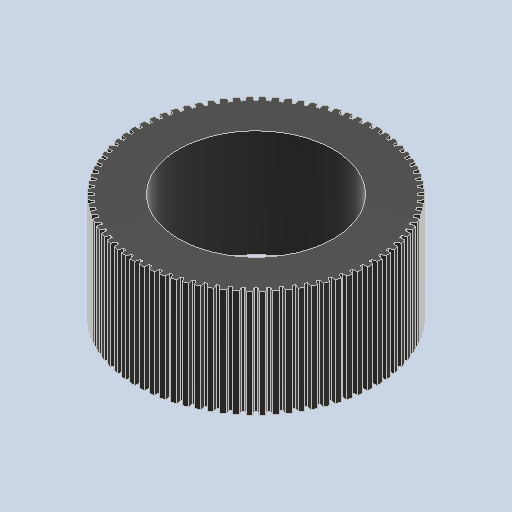
# Autodesk Inventor part: タミヤダンパー3
Saved by Autodesk Inventor 2023 (Build 270158030, 158C)
## iProperties
Part Number: タミヤダンパー3
Material: アセタール樹脂、黒
Document SubType Name: Modeling
Designer: 雪村
Density: 1.425 g/cm^3
Appearance: 滑らか - 黒
Mass: 0.276107 g
Surface Area: 4.29277 cm^2
Volume: 0.193759 cm^3
Author: 雪村
Autodesk Inventor part; units mm, degrees
ref_plane "YZ Plane" through (0, 0, 0) normal (1, 0, 0) x (0, 1, 0)
ref_plane "XZ Plane" through (0, 0, 0) normal (0, 1, 0) x (-1, 0, 0)
ref_plane "XY Plane" through (0, 0, 0) normal (0, 0, 1) x (1, 0, 0)
sketch "スケッチ1" plane through (0, 0, 0) normal (0, 0, 1) x (1, 0, 0)
  circle A0 centre (0, 0) radius 5
  dimension "d0" = 10
  constraints: 1 centre point, 1 coincident
  measures "d0" diameter of A0
extrude "押し出し1" add sketch "スケッチ1" along normal blind 4.5
sketch "スケッチ2" plane through (0, 0, 4.5) normal (0, 0, 1) x (1, 0, 0)
  circle A0 centre (0, 0) radius 3.25
  dimension "d3" = 6.5
  constraints: 1 centre point, 1 coincident
  measures "d3" diameter of A0
extrude "押し出し2" cut sketch "スケッチ2" against normal through all
sketch "スケッチ3" plane through (0, 0, 4.5) normal (0, 0, 1) x (1, 0, 0)
  arc A0 (0.0974, 4.9991) -> (-0.0974, 4.9991) centre (0, 0) ccw
  arc A1 (0.05, 4.8047) -> (-0.05, 4.8047) centre (0, 0) ccw
  line L0 (0.05, 4.8047) -> (0.0974, 4.9991)
  line L1 (-0.05, 4.8047) -> (-0.0974, 4.9991)
  line L2 (0, 4.9011) -> (0, 0)
  line L3 (-0.4268, 4.786) -> (-0.4893, 4.976)
  arc A2 (-0.2952, 4.9913) -> (-0.4893, 4.976) centre (0, 0) ccw
  line L4 (-0.3271, 4.7939) -> (-0.2952, 4.9913)
  arc A3 (-0.3271, 4.7939) -> (-0.4268, 4.786) centre (0, 0) ccw
  line L5 (-0.801, 4.7378) -> (-0.8782, 4.9223)
  arc A4 (-0.6859, 4.9527) -> (-0.8782, 4.9223) centre (0, 0) ccw
  line L6 (-0.7022, 4.7534) -> (-0.6859, 4.9527)
  arc A5 (-0.7022, 4.7534) -> (-0.801, 4.7378) centre (0, 0) ccw
  line L7 (-1.1703, 4.6603) -> (-1.2617, 4.8382)
  arc A6 (-1.0723, 4.8837) -> (-1.2617, 4.8382) centre (0, 0) ccw
  line L8 (-1.073, 4.6837) -> (-1.0723, 4.8837)
  arc A7 (-1.073, 4.6837) -> (-1.1703, 4.6603) centre (0, 0) ccw
  line L9 (-1.5323, 4.5541) -> (-1.6374, 4.7243)
  arc A8 (-1.4522, 4.7845) -> (-1.6374, 4.7243) centre (0, 0) ccw
  line L10 (-1.4372, 4.585) -> (-1.4522, 4.7845)
  arc A9 (-1.4372, 4.585) -> (-1.5323, 4.5541) centre (0, 0) ccw
  line L11 (-1.8849, 4.4199) -> (-2.003, 4.5813)
  arc A10 (-1.8231, 4.6558) -> (-2.003, 4.5813) centre (0, 0) ccw
  line L12 (-1.7925, 4.4581) -> (-1.8231, 4.6558)
  arc A11 (-1.7925, 4.4581) -> (-1.8849, 4.4199) centre (0, 0) ccw
  line L13 (-2.2259, 4.2584) -> (-2.3563, 4.41)
  arc A12 (-2.1828, 4.4984) -> (-2.3563, 4.41) centre (0, 0) ccw
  line L14 (-2.1368, 4.3038) -> (-2.1828, 4.4984)
  arc A13 (-2.1368, 4.3038) -> (-2.2259, 4.2584) centre (0, 0) ccw
  line L15 (-2.5531, 4.0706) -> (-2.695, 4.2115)
  arc A14 (-2.529, 4.3133) -> (-2.695, 4.2115) centre (0, 0) ccw
  line L16 (-2.4678, 4.1228) -> (-2.529, 4.3133)
  arc A15 (-2.4678, 4.1228) -> (-2.5531, 4.0706) centre (0, 0) ccw
  line L17 (-2.8646, 3.8577) -> (-3.0171, 3.9871)
  arc A16 (-2.8596, 4.1015) -> (-3.0171, 3.9871) centre (0, 0) ccw
  line L18 (-2.7837, 3.9165) -> (-2.8596, 4.1015)
  arc A17 (-2.7837, 3.9165) -> (-2.8646, 3.8577) centre (0, 0) ccw
  line L19 (-3.1584, 3.6211) -> (-3.3207, 3.7381)
  arc A18 (-3.1726, 3.8645) -> (-3.3207, 3.7381) centre (0, 0) ccw
  line L20 (-3.0824, 3.686) -> (-3.1726, 3.8645)
  arc A19 (-3.0824, 3.686) -> (-3.1584, 3.6211) centre (0, 0) ccw
  line L21 (-3.4328, 3.3621) -> (-3.6037, 3.466)
  arc A20 (-3.466, 3.6037) -> (-3.6037, 3.466) centre (0, 0) ccw
  line L22 (-3.3621, 3.4328) -> (-3.466, 3.6037)
  arc A21 (-3.3621, 3.4328) -> (-3.4328, 3.3621) centre (0, 0) ccw
  line L23 (-3.686, 3.0824) -> (-3.8645, 3.1726)
  arc A22 (-3.7381, 3.3207) -> (-3.8645, 3.1726) centre (0, 0) ccw
  line L24 (-3.6211, 3.1584) -> (-3.7381, 3.3207)
  arc A23 (-3.6211, 3.1584) -> (-3.686, 3.0824) centre (0, 0) ccw
  line L25 (-3.9165, 2.7837) -> (-4.1015, 2.8596)
  arc A24 (-3.9871, 3.0171) -> (-4.1015, 2.8596) centre (0, 0) ccw
  line L26 (-3.8577, 2.8646) -> (-3.9871, 3.0171)
  arc A25 (-3.8577, 2.8646) -> (-3.9165, 2.7837) centre (0, 0) ccw
  line L27 (-4.1228, 2.4678) -> (-4.3133, 2.529)
  arc A26 (-4.2115, 2.695) -> (-4.3133, 2.529) centre (0, 0) ccw
  line L28 (-4.0706, 2.5531) -> (-4.2115, 2.695)
  arc A27 (-4.0706, 2.5531) -> (-4.1228, 2.4678) centre (0, 0) ccw
  line L29 (-4.3038, 2.1368) -> (-4.4984, 2.1828)
  arc A28 (-4.41, 2.3563) -> (-4.4984, 2.1828) centre (0, 0) ccw
  line L30 (-4.2584, 2.2259) -> (-4.41, 2.3563)
  arc A29 (-4.2584, 2.2259) -> (-4.3038, 2.1368) centre (0, 0) ccw
  line L31 (-4.4581, 1.7925) -> (-4.6558, 1.8231)
  arc A30 (-4.5813, 2.003) -> (-4.6558, 1.8231) centre (0, 0) ccw
  line L32 (-4.4199, 1.8849) -> (-4.5813, 2.003)
  arc A31 (-4.4199, 1.8849) -> (-4.4581, 1.7925) centre (0, 0) ccw
  line L33 (-4.585, 1.4372) -> (-4.7845, 1.4522)
  arc A32 (-4.7243, 1.6374) -> (-4.7845, 1.4522) centre (0, 0) ccw
  line L34 (-4.5541, 1.5323) -> (-4.7243, 1.6374)
  arc A33 (-4.5541, 1.5323) -> (-4.585, 1.4372) centre (0, 0) ccw
  line L35 (-4.6837, 1.073) -> (-4.8837, 1.0723)
  arc A34 (-4.8382, 1.2617) -> (-4.8837, 1.0723) centre (0, 0) ccw
  line L36 (-4.6603, 1.1703) -> (-4.8382, 1.2617)
  arc A35 (-4.6603, 1.1703) -> (-4.6837, 1.073) centre (0, 0) ccw
  line L37 (-4.7534, 0.7022) -> (-4.9527, 0.6859)
  arc A36 (-4.9223, 0.8782) -> (-4.9527, 0.6859) centre (0, 0) ccw
  line L38 (-4.7378, 0.801) -> (-4.9223, 0.8782)
  arc A37 (-4.7378, 0.801) -> (-4.7534, 0.7022) centre (0, 0) ccw
  line L39 (-4.7939, 0.3271) -> (-4.9913, 0.2952)
  arc A38 (-4.976, 0.4893) -> (-4.9913, 0.2952) centre (0, 0) ccw
  line L40 (-4.786, 0.4268) -> (-4.976, 0.4893)
  arc A39 (-4.786, 0.4268) -> (-4.7939, 0.3271) centre (0, 0) ccw
  line L41 (-4.8047, -0.05) -> (-4.9991, -0.0974)
  arc A40 (-4.9991, 0.0974) -> (-4.9991, -0.0974) centre (0, 0) ccw
  line L42 (-4.8047, 0.05) -> (-4.9991, 0.0974)
  arc A41 (-4.8047, 0.05) -> (-4.8047, -0.05) centre (0, 0) ccw
  line L43 (-4.786, -0.4268) -> (-4.976, -0.4893)
  arc A42 (-4.9913, -0.2952) -> (-4.976, -0.4893) centre (0, 0) ccw
  line L44 (-4.7939, -0.3271) -> (-4.9913, -0.2952)
  arc A43 (-4.7939, -0.3271) -> (-4.786, -0.4268) centre (0, 0) ccw
  line L45 (-4.7378, -0.801) -> (-4.9223, -0.8782)
  arc A44 (-4.9527, -0.6859) -> (-4.9223, -0.8782) centre (0, 0) ccw
  line L46 (-4.7534, -0.7022) -> (-4.9527, -0.6859)
  arc A45 (-4.7534, -0.7022) -> (-4.7378, -0.801) centre (0, 0) ccw
  line L47 (-4.6603, -1.1703) -> (-4.8382, -1.2617)
  arc A46 (-4.8837, -1.0723) -> (-4.8382, -1.2617) centre (0, 0) ccw
  line L48 (-4.6837, -1.073) -> (-4.8837, -1.0723)
  arc A47 (-4.6837, -1.073) -> (-4.6603, -1.1703) centre (0, 0) ccw
  line L49 (-4.5541, -1.5323) -> (-4.7243, -1.6374)
  arc A48 (-4.7845, -1.4522) -> (-4.7243, -1.6374) centre (0, 0) ccw
  line L50 (-4.585, -1.4372) -> (-4.7845, -1.4522)
  arc A49 (-4.585, -1.4372) -> (-4.5541, -1.5323) centre (0, 0) ccw
  line L51 (-4.4199, -1.8849) -> (-4.5813, -2.003)
  arc A50 (-4.6558, -1.8231) -> (-4.5813, -2.003) centre (0, 0) ccw
  line L52 (-4.4581, -1.7925) -> (-4.6558, -1.8231)
  arc A51 (-4.4581, -1.7925) -> (-4.4199, -1.8849) centre (0, 0) ccw
  line L53 (-4.2584, -2.2259) -> (-4.41, -2.3563)
  arc A52 (-4.4984, -2.1828) -> (-4.41, -2.3563) centre (0, 0) ccw
  line L54 (-4.3038, -2.1368) -> (-4.4984, -2.1828)
  arc A53 (-4.3038, -2.1368) -> (-4.2584, -2.2259) centre (0, 0) ccw
  line L55 (-4.0706, -2.5531) -> (-4.2115, -2.695)
  arc A54 (-4.3133, -2.529) -> (-4.2115, -2.695) centre (0, 0) ccw
  line L56 (-4.1228, -2.4678) -> (-4.3133, -2.529)
  arc A55 (-4.1228, -2.4678) -> (-4.0706, -2.5531) centre (0, 0) ccw
  line L57 (-3.8577, -2.8646) -> (-3.9871, -3.0171)
  arc A56 (-4.1015, -2.8596) -> (-3.9871, -3.0171) centre (0, 0) ccw
  line L58 (-3.9165, -2.7837) -> (-4.1015, -2.8596)
  arc A57 (-3.9165, -2.7837) -> (-3.8577, -2.8646) centre (0, 0) ccw
  line L59 (-3.6211, -3.1584) -> (-3.7381, -3.3207)
  arc A58 (-3.8645, -3.1726) -> (-3.7381, -3.3207) centre (0, 0) ccw
  line L60 (-3.686, -3.0824) -> (-3.8645, -3.1726)
  arc A59 (-3.686, -3.0824) -> (-3.6211, -3.1584) centre (0, 0) ccw
  line L61 (-3.3621, -3.4328) -> (-3.466, -3.6037)
  arc A60 (-3.6037, -3.466) -> (-3.466, -3.6037) centre (0, 0) ccw
  line L62 (-3.4328, -3.3621) -> (-3.6037, -3.466)
  arc A61 (-3.4328, -3.3621) -> (-3.3621, -3.4328) centre (0, 0) ccw
  line L63 (-3.0824, -3.686) -> (-3.1726, -3.8645)
  arc A62 (-3.3207, -3.7381) -> (-3.1726, -3.8645) centre (0, 0) ccw
  line L64 (-3.1584, -3.6211) -> (-3.3207, -3.7381)
  arc A63 (-3.1584, -3.6211) -> (-3.0824, -3.686) centre (0, 0) ccw
  line L65 (-2.7837, -3.9165) -> (-2.8596, -4.1015)
  arc A64 (-3.0171, -3.9871) -> (-2.8596, -4.1015) centre (0, 0) ccw
  line L66 (-2.8646, -3.8577) -> (-3.0171, -3.9871)
  arc A65 (-2.8646, -3.8577) -> (-2.7837, -3.9165) centre (0, 0) ccw
  line L67 (-2.4678, -4.1228) -> (-2.529, -4.3133)
  arc A66 (-2.695, -4.2115) -> (-2.529, -4.3133) centre (0, 0) ccw
  line L68 (-2.5531, -4.0706) -> (-2.695, -4.2115)
  arc A67 (-2.5531, -4.0706) -> (-2.4678, -4.1228) centre (0, 0) ccw
  line L69 (-2.1368, -4.3038) -> (-2.1828, -4.4984)
  arc A68 (-2.3563, -4.41) -> (-2.1828, -4.4984) centre (0, 0) ccw
  line L70 (-2.2259, -4.2584) -> (-2.3563, -4.41)
  arc A69 (-2.2259, -4.2584) -> (-2.1368, -4.3038) centre (0, 0) ccw
  line L71 (-1.7925, -4.4581) -> (-1.8231, -4.6558)
  arc A70 (-2.003, -4.5813) -> (-1.8231, -4.6558) centre (0, 0) ccw
  line L72 (-1.8849, -4.4199) -> (-2.003, -4.5813)
  arc A71 (-1.8849, -4.4199) -> (-1.7925, -4.4581) centre (0, 0) ccw
  line L73 (-1.4372, -4.585) -> (-1.4522, -4.7845)
  arc A72 (-1.6374, -4.7243) -> (-1.4522, -4.7845) centre (0, 0) ccw
  line L74 (-1.5323, -4.5541) -> (-1.6374, -4.7243)
  arc A73 (-1.5323, -4.5541) -> (-1.4372, -4.585) centre (0, 0) ccw
  line L75 (-1.073, -4.6837) -> (-1.0723, -4.8837)
  arc A74 (-1.2617, -4.8382) -> (-1.0723, -4.8837) centre (0, 0) ccw
  line L76 (-1.1703, -4.6603) -> (-1.2617, -4.8382)
  arc A75 (-1.1703, -4.6603) -> (-1.073, -4.6837) centre (0, 0) ccw
  line L77 (-0.7022, -4.7534) -> (-0.6859, -4.9527)
  arc A76 (-0.8782, -4.9223) -> (-0.6859, -4.9527) centre (0, 0) ccw
  line L78 (-0.801, -4.7378) -> (-0.8782, -4.9223)
  arc A77 (-0.801, -4.7378) -> (-0.7022, -4.7534) centre (0, 0) ccw
  line L79 (-0.3271, -4.7939) -> (-0.2952, -4.9913)
  arc A78 (-0.4893, -4.976) -> (-0.2952, -4.9913) centre (0, 0) ccw
  line L80 (-0.4268, -4.786) -> (-0.4893, -4.976)
  arc A79 (-0.4268, -4.786) -> (-0.3271, -4.7939) centre (0, 0) ccw
  line L81 (0.05, -4.8047) -> (0.0974, -4.9991)
  arc A80 (-0.0974, -4.9991) -> (0.0974, -4.9991) centre (0, 0) ccw
  line L82 (-0.05, -4.8047) -> (-0.0974, -4.9991)
  arc A81 (-0.05, -4.8047) -> (0.05, -4.8047) centre (0, 0) ccw
  line L83 (0.4268, -4.786) -> (0.4893, -4.976)
  arc A82 (0.2952, -4.9913) -> (0.4893, -4.976) centre (0, 0) ccw
  line L84 (0.3271, -4.7939) -> (0.2952, -4.9913)
  arc A83 (0.3271, -4.7939) -> (0.4268, -4.786) centre (0, 0) ccw
  line L85 (0.801, -4.7378) -> (0.8782, -4.9223)
  arc A84 (0.6859, -4.9527) -> (0.8782, -4.9223) centre (0, 0) ccw
  line L86 (0.7022, -4.7534) -> (0.6859, -4.9527)
  arc A85 (0.7022, -4.7534) -> (0.801, -4.7378) centre (0, 0) ccw
  line L87 (1.1703, -4.6603) -> (1.2617, -4.8382)
  arc A86 (1.0723, -4.8837) -> (1.2617, -4.8382) centre (0, 0) ccw
  line L88 (1.073, -4.6837) -> (1.0723, -4.8837)
  arc A87 (1.073, -4.6837) -> (1.1703, -4.6603) centre (0, 0) ccw
  line L89 (1.5323, -4.5541) -> (1.6374, -4.7243)
  arc A88 (1.4522, -4.7845) -> (1.6374, -4.7243) centre (0, 0) ccw
  line L90 (1.4372, -4.585) -> (1.4522, -4.7845)
  arc A89 (1.4372, -4.585) -> (1.5323, -4.5541) centre (0, 0) ccw
  line L91 (1.8849, -4.4199) -> (2.003, -4.5813)
  arc A90 (1.8231, -4.6558) -> (2.003, -4.5813) centre (0, 0) ccw
  line L92 (1.7925, -4.4581) -> (1.8231, -4.6558)
  arc A91 (1.7925, -4.4581) -> (1.8849, -4.4199) centre (0, 0) ccw
  line L93 (2.2259, -4.2584) -> (2.3563, -4.41)
  arc A92 (2.1828, -4.4984) -> (2.3563, -4.41) centre (0, 0) ccw
  line L94 (2.1368, -4.3038) -> (2.1828, -4.4984)
  arc A93 (2.1368, -4.3038) -> (2.2259, -4.2584) centre (0, 0) ccw
  line L95 (2.5531, -4.0706) -> (2.695, -4.2115)
  arc A94 (2.529, -4.3133) -> (2.695, -4.2115) centre (0, 0) ccw
  line L96 (2.4678, -4.1228) -> (2.529, -4.3133)
  arc A95 (2.4678, -4.1228) -> (2.5531, -4.0706) centre (0, 0) ccw
  line L97 (2.8646, -3.8577) -> (3.0171, -3.9871)
  arc A96 (2.8596, -4.1015) -> (3.0171, -3.9871) centre (0, 0) ccw
  line L98 (2.7837, -3.9165) -> (2.8596, -4.1015)
  arc A97 (2.7837, -3.9165) -> (2.8646, -3.8577) centre (0, 0) ccw
  line L99 (3.1584, -3.6211) -> (3.3207, -3.7381)
  arc A98 (3.1726, -3.8645) -> (3.3207, -3.7381) centre (0, 0) ccw
  line L100 (3.0824, -3.686) -> (3.1726, -3.8645)
  arc A99 (3.0824, -3.686) -> (3.1584, -3.6211) centre (0, 0) ccw
  line L101 (3.4328, -3.3621) -> (3.6037, -3.466)
  arc A100 (3.466, -3.6037) -> (3.6037, -3.466) centre (0, 0) ccw
  line L102 (3.3621, -3.4328) -> (3.466, -3.6037)
  arc A101 (3.3621, -3.4328) -> (3.4328, -3.3621) centre (0, 0) ccw
  line L103 (3.686, -3.0824) -> (3.8645, -3.1726)
  arc A102 (3.7381, -3.3207) -> (3.8645, -3.1726) centre (0, 0) ccw
  line L104 (3.6211, -3.1584) -> (3.7381, -3.3207)
  arc A103 (3.6211, -3.1584) -> (3.686, -3.0824) centre (0, 0) ccw
  line L105 (3.9165, -2.7837) -> (4.1015, -2.8596)
  arc A104 (3.9871, -3.0171) -> (4.1015, -2.8596) centre (0, 0) ccw
  line L106 (3.8577, -2.8646) -> (3.9871, -3.0171)
  arc A105 (3.8577, -2.8646) -> (3.9165, -2.7837) centre (0, 0) ccw
  line L107 (4.1228, -2.4678) -> (4.3133, -2.529)
  arc A106 (4.2115, -2.695) -> (4.3133, -2.529) centre (0, 0) ccw
  line L108 (4.0706, -2.5531) -> (4.2115, -2.695)
  arc A107 (4.0706, -2.5531) -> (4.1228, -2.4678) centre (0, 0) ccw
  line L109 (4.3038, -2.1368) -> (4.4984, -2.1828)
  arc A108 (4.41, -2.3563) -> (4.4984, -2.1828) centre (0, 0) ccw
  line L110 (4.2584, -2.2259) -> (4.41, -2.3563)
  arc A109 (4.2584, -2.2259) -> (4.3038, -2.1368) centre (0, 0) ccw
  line L111 (4.4581, -1.7925) -> (4.6558, -1.8231)
  arc A110 (4.5813, -2.003) -> (4.6558, -1.8231) centre (0, 0) ccw
  line L112 (4.4199, -1.8849) -> (4.5813, -2.003)
  arc A111 (4.4199, -1.8849) -> (4.4581, -1.7925) centre (0, 0) ccw
  line L113 (4.585, -1.4372) -> (4.7845, -1.4522)
  arc A112 (4.7243, -1.6374) -> (4.7845, -1.4522) centre (0, 0) ccw
  line L114 (4.5541, -1.5323) -> (4.7243, -1.6374)
  arc A113 (4.5541, -1.5323) -> (4.585, -1.4372) centre (0, 0) ccw
  line L115 (4.6837, -1.073) -> (4.8837, -1.0723)
  arc A114 (4.8382, -1.2617) -> (4.8837, -1.0723) centre (0, 0) ccw
  line L116 (4.6603, -1.1703) -> (4.8382, -1.2617)
  arc A115 (4.6603, -1.1703) -> (4.6837, -1.073) centre (0, 0) ccw
  line L117 (4.7534, -0.7022) -> (4.9527, -0.6859)
  arc A116 (4.9223, -0.8782) -> (4.9527, -0.6859) centre (0, 0) ccw
  line L118 (4.7378, -0.801) -> (4.9223, -0.8782)
  arc A117 (4.7378, -0.801) -> (4.7534, -0.7022) centre (0, 0) ccw
  line L119 (4.7939, -0.3271) -> (4.9913, -0.2952)
  arc A118 (4.976, -0.4893) -> (4.9913, -0.2952) centre (0, 0) ccw
  line L120 (4.786, -0.4268) -> (4.976, -0.4893)
  arc A119 (4.786, -0.4268) -> (4.7939, -0.3271) centre (0, 0) ccw
  line L121 (4.8047, 0.05) -> (4.9991, 0.0974)
  arc A120 (4.9991, -0.0974) -> (4.9991, 0.0974) centre (0, 0) ccw
  line L122 (4.8047, -0.05) -> (4.9991, -0.0974)
  arc A121 (4.8047, -0.05) -> (4.8047, 0.05) centre (0, 0) ccw
  line L123 (4.786, 0.4268) -> (4.976, 0.4893)
  arc A122 (4.9913, 0.2952) -> (4.976, 0.4893) centre (0, 0) ccw
  line L124 (4.7939, 0.3271) -> (4.9913, 0.2952)
  arc A123 (4.7939, 0.3271) -> (4.786, 0.4268) centre (0, 0) ccw
  line L125 (4.7378, 0.801) -> (4.9223, 0.8782)
  arc A124 (4.9527, 0.6859) -> (4.9223, 0.8782) centre (0, 0) ccw
  line L126 (4.7534, 0.7022) -> (4.9527, 0.6859)
  arc A125 (4.7534, 0.7022) -> (4.7378, 0.801) centre (0, 0) ccw
  line L127 (4.6603, 1.1703) -> (4.8382, 1.2617)
  arc A126 (4.8837, 1.0723) -> (4.8382, 1.2617) centre (0, 0) ccw
  line L128 (4.6837, 1.073) -> (4.8837, 1.0723)
  arc A127 (4.6837, 1.073) -> (4.6603, 1.1703) centre (0, 0) ccw
  line L129 (4.5541, 1.5323) -> (4.7243, 1.6374)
  arc A128 (4.7845, 1.4522) -> (4.7243, 1.6374) centre (0, 0) ccw
  line L130 (4.585, 1.4372) -> (4.7845, 1.4522)
  arc A129 (4.585, 1.4372) -> (4.5541, 1.5323) centre (0, 0) ccw
  line L131 (4.4199, 1.8849) -> (4.5813, 2.003)
  arc A130 (4.6558, 1.8231) -> (4.5813, 2.003) centre (0, 0) ccw
  line L132 (4.4581, 1.7925) -> (4.6558, 1.8231)
  arc A131 (4.4581, 1.7925) -> (4.4199, 1.8849) centre (0, 0) ccw
  line L133 (4.2584, 2.2259) -> (4.41, 2.3563)
  arc A132 (4.4984, 2.1828) -> (4.41, 2.3563) centre (0, 0) ccw
  line L134 (4.3038, 2.1368) -> (4.4984, 2.1828)
  arc A133 (4.3038, 2.1368) -> (4.2584, 2.2259) centre (0, 0) ccw
  line L135 (4.0706, 2.5531) -> (4.2115, 2.695)
  arc A134 (4.3133, 2.529) -> (4.2115, 2.695) centre (0, 0) ccw
  line L136 (4.1228, 2.4678) -> (4.3133, 2.529)
  arc A135 (4.1228, 2.4678) -> (4.0706, 2.5531) centre (0, 0) ccw
  line L137 (3.8577, 2.8646) -> (3.9871, 3.0171)
  arc A136 (4.1015, 2.8596) -> (3.9871, 3.0171) centre (0, 0) ccw
  line L138 (3.9165, 2.7837) -> (4.1015, 2.8596)
  arc A137 (3.9165, 2.7837) -> (3.8577, 2.8646) centre (0, 0) ccw
  line L139 (3.6211, 3.1584) -> (3.7381, 3.3207)
  arc A138 (3.8645, 3.1726) -> (3.7381, 3.3207) centre (0, 0) ccw
  line L140 (3.686, 3.0824) -> (3.8645, 3.1726)
  arc A139 (3.686, 3.0824) -> (3.6211, 3.1584) centre (0, 0) ccw
  line L141 (3.3621, 3.4328) -> (3.466, 3.6037)
  arc A140 (3.6037, 3.466) -> (3.466, 3.6037) centre (0, 0) ccw
  line L142 (3.4328, 3.3621) -> (3.6037, 3.466)
  arc A141 (3.4328, 3.3621) -> (3.3621, 3.4328) centre (0, 0) ccw
  line L143 (3.0824, 3.686) -> (3.1726, 3.8645)
  arc A142 (3.3207, 3.7381) -> (3.1726, 3.8645) centre (0, 0) ccw
  line L144 (3.1584, 3.6211) -> (3.3207, 3.7381)
  arc A143 (3.1584, 3.6211) -> (3.0824, 3.686) centre (0, 0) ccw
  line L145 (2.7837, 3.9165) -> (2.8596, 4.1015)
  arc A144 (3.0171, 3.9871) -> (2.8596, 4.1015) centre (0, 0) ccw
  line L146 (2.8646, 3.8577) -> (3.0171, 3.9871)
  arc A145 (2.8646, 3.8577) -> (2.7837, 3.9165) centre (0, 0) ccw
  line L147 (2.4678, 4.1228) -> (2.529, 4.3133)
  arc A146 (2.695, 4.2115) -> (2.529, 4.3133) centre (0, 0) ccw
  line L148 (2.5531, 4.0706) -> (2.695, 4.2115)
  arc A147 (2.5531, 4.0706) -> (2.4678, 4.1228) centre (0, 0) ccw
  line L149 (2.1368, 4.3038) -> (2.1828, 4.4984)
  arc A148 (2.3563, 4.41) -> (2.1828, 4.4984) centre (0, 0) ccw
  line L150 (2.2259, 4.2584) -> (2.3563, 4.41)
  arc A149 (2.2259, 4.2584) -> (2.1368, 4.3038) centre (0, 0) ccw
  line L151 (1.7925, 4.4581) -> (1.8231, 4.6558)
  arc A150 (2.003, 4.5813) -> (1.8231, 4.6558) centre (0, 0) ccw
  line L152 (1.8849, 4.4199) -> (2.003, 4.5813)
  arc A151 (1.8849, 4.4199) -> (1.7925, 4.4581) centre (0, 0) ccw
  line L153 (1.4372, 4.585) -> (1.4522, 4.7845)
  arc A152 (1.6374, 4.7243) -> (1.4522, 4.7845) centre (0, 0) ccw
  line L154 (1.5323, 4.5541) -> (1.6374, 4.7243)
  arc A153 (1.5323, 4.5541) -> (1.4372, 4.585) centre (0, 0) ccw
  line L155 (1.073, 4.6837) -> (1.0723, 4.8837)
  arc A154 (1.2617, 4.8382) -> (1.0723, 4.8837) centre (0, 0) ccw
  line L156 (1.1703, 4.6603) -> (1.2617, 4.8382)
  arc A155 (1.1703, 4.6603) -> (1.073, 4.6837) centre (0, 0) ccw
  line L157 (0.7022, 4.7534) -> (0.6859, 4.9527)
  arc A156 (0.8782, 4.9223) -> (0.6859, 4.9527) centre (0, 0) ccw
  line L158 (0.801, 4.7378) -> (0.8782, 4.9223)
  arc A157 (0.801, 4.7378) -> (0.7022, 4.7534) centre (0, 0) ccw
  line L159 (0.3271, 4.7939) -> (0.2952, 4.9913)
  arc A158 (0.4893, 4.976) -> (0.2952, 4.9913) centre (0, 0) ccw
  line L160 (0.4268, 4.786) -> (0.4893, 4.976)
  arc A159 (0.4268, 4.786) -> (0.3271, 4.7939) centre (0, 0) ccw
  dimension "d6" = 0.2
  dimension "d7" = 0.2
  dimension "d8" = 0.1
  dimension "d9" = 9.61
  dimension "d10" = 0.05
  dimension "d13" = 360
  constraints: 322 end point, 320 point on circle, 160 centre point, 81 coincident, 1 vertical, 802 other
  measures "d6" distance of L1.start L1.end
  measures "d7" distance of L0.start L0.end
  measures "d8" distance of L0.start L1.start
  measures "d9" diameter of A1
  measures "d10" distance from line of L2 L1.start
extrude "押し出し3" cut sketch "スケッチ3" against normal through all
equation "\"d7\" = d6"
